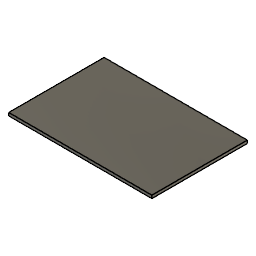
coil housing bottom and top plate (Autodesk Fusion 360 design; units mm, degrees)
part number: 2026-08-05-15-10-08-862
Autodesk Fusion 360 part; units mm, degrees
sketch "Sketch1" plane through (0, 0, 0) normal (0, 0, 1) x (1, 0, 0)
  line L0 (152.4, 101.6) -> (-152.4, 101.6)
  line L1 (-152.4, 101.6) -> (-152.4, -101.6)
  line L2 (-152.4, -101.6) -> (152.4, -101.6)
  line L3 (152.4, -101.6) -> (152.4, 101.6)
  line L4 (152.4, 101.6) -> (-152.4, -101.6) construction
  line L5 (-152.4, 101.6) -> (152.4, -101.6) construction
  dimension "d1" = 304.8
  dimension "d2" = 203.2
  constraint horizontal L0
  constraint perpendicular L0 L1
  constraint parallel L0 L2
  constraint parallel L1 L3
  constraint coincident L4 origin
  constraint coincident L5 origin
  measures "d1" distance of L1.end L2.end
  measures "d2" distance of L0.end L1.end
extrude "Extrude1" add sketch "Sketch1" along normal blind 6.35
